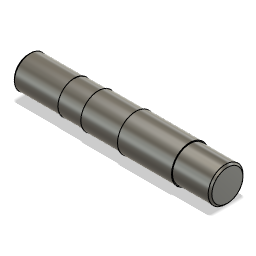
FUSHION (Autodesk Fusion 360 design; units mm, degrees)
Autodesk Fusion 360 part; units mm, degrees
sketch "Sketch1" plane through (0, 0, 0) normal (0, 1, 0) x (1, 0, 0)
  line L0 (0, 0) -> (50, 0)
  line L1 (50, 0) -> (50, -17.5)
  line L2 (0, 0) -> (0, -17.5)
  line L3 (0, -17.5) -> (50, -17.5)
  line L4 (50, 0) -> (76, 0)
  line L5 (76, 0) -> (76, -18)
  line L6 (76, -18) -> (50, -18)
  line L7 (50, 0) -> (50, -18)
  line L8 (76, 0) -> (117, 0)
  line L9 (117, 0) -> (117, -19)
  line L10 (76, 0) -> (76, -19)
  line L11 (76, -19) -> (117, -19)
  line L12 (117, 0) -> (176, 0)
  line L13 (117, 0) -> (117, -20)
  line L14 (117, -20) -> (176, -20)
  line L15 (176, 0) -> (176, -20)
  line L16 (176, 0) -> (217, 0)
  line L17 (217, 0) -> (217, -19)
  line L18 (217, -19) -> (176, -19)
  dimension "d1" = 50
  dimension "d2" = 17.5
  dimension "d3" = 17.5
  dimension "d4" = 26
  dimension "d5" = 18
  dimension "d6" = 26
  dimension "d7" = 41
  dimension "d8" = 19
  dimension "d9" = 19
  dimension "d10" = 59
  dimension "d11" = 20
  dimension "d12" = 59
  dimension "d13" = 41
  dimension "d14" = 19
  constraint coincident L0.start L2.start
  constraint horizontal L0
  constraint perpendicular L0 L1
  constraint vertical L2
  constraint perpendicular L1 L4
  constraint perpendicular L4 L5
  constraint perpendicular L5 L6
  constraint perpendicular L5 L8
  constraint perpendicular L8 L9
  constraint perpendicular L8 L10
  constraint perpendicular L9 L12
  constraint perpendicular L8 L13
  constraint perpendicular L13 L14
  constraint perpendicular L15 L16
  constraint perpendicular L16 L17
  constraint coincident L15 L18.end
  constraint perpendicular L15 L18
  measures "d1" distance of L0.start L0.end
  measures "d2" distance of L0.end L1.end
  measures "d3" distance of L0.start L2.end
  measures "d4" distance of L0.end L4.end
  measures "d5" distance of L4.end L5.end
  measures "d6" distance of L5.end L6.end
  measures "d7" distance of L4.end L8.end
  measures "d8" distance of L8.end L9.end
  measures "d9" distance of L4.end L10.end
  measures "d10" distance of L8.end L12.end
  measures "d11" distance of L8.end L13.end
  measures "d12" distance of L13.end L14.end
  measures "d13" distance of L12.end L16.end
  measures "d14" distance of L16.end L17.end
revolve "Revolve1" add sketch "Sketch1" angle 360 about axis through (76, 0, 0) along (1, 0, 0)
sketch "Sketch2" plane through (0, 0, 0) normal (0, 0, 1) x (1, 0, 0)
  line L0 (11.2338, -5, -17.8) -> (36.938, -5, -17.8)
  arc A0 through (36.938, -5, -17.8) (41.938, 0, -17.8) (36.938, 5, -17.8)
  line L1 (36.938, 5, -17.8) -> (11.2338, 5, -17.8)
  arc A1 through (11.2338, 5, -17.8) (6.2338, 0, -17.8) (11.2338, -5, -17.8)
  line L2 (11.2338, 0, -17.8) -> (36.938, 0, -17.8) construction
  dimension "d16" = 10
sketch "Sketch3" plane through (0, 0, 0) normal (0, 0, 1) x (1, 0, 0)
sketch "Sketch4" plane through (0, 0, 0) normal (0, 0, 1) x (1, 0, 0)
sketch "Sketch5" plane through (0, 0, 0) normal (0, 0, 1) x (1, 0, 0)
extrude "Extrude1" cut sketch "Sketch2" along normal blind 5.5 contours L0 A0 L1 A1 in plane through (0, 0, -17.8) normal (0, 0, 1)
sketch "Sketch6" plane through (0, 0, 0) normal (0, 0, 1) x (1, 0, 0)
  line L0 (164.1003, 6.8616, -20.1) -> (128.1003, 6.8616, -20.1)
  arc A0 through (128.1003, 6.8616, -20.1) (122.1003, 0.8616, -20.1) (128.1003, -5.1384, -20.1)
  line L1 (128.1003, -5.1384, -20.1) -> (164.1003, -5.1384, -20.1)
  arc A1 through (164.1003, -5.1384, -20.1) (170.1003, 0.8616, -20.1) (164.1003, 6.8616, -20.1)
  line L2 (164.1003, 0.8616, -20.1) -> (128.1003, 0.8616, -20.1) construction
  dimension "d19" = 12
  dimension "d20" = 36
extrude "Extrude2" cut sketch "Sketch6" along normal blind 5.5 contours L0 A0 L1 A1 in plane through (0, 0, -20.1) normal (0, 0, 1)
chamfer "Chamfer1" distance 2 angle 45 1 edges at (217, -6.8707, -17.7142)
chamfer "Chamfer2" distance 2 angle 45 1 edges at (0, -6.3283, -16.3157)
